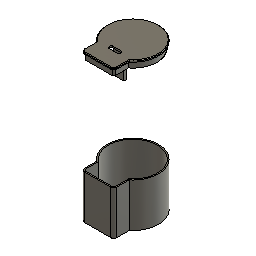
Co2SensorEnclosure (Autodesk Fusion 360 design; units mm, degrees)
Autodesk Fusion 360 part; units mm, degrees
sketch "Sketch1" plane through (0, 0, 0) normal (0, 1, 0) x (1, 0, 0)
  line L0 (0, 19) -> (0, -26.75) construction
  line L1 (0, -26.75) -> (11.5, -26.75) construction
  line L2 (10.5, -26.75) -> (-10.5, -26.75) construction
  line L3 (-11.5, -25.75) -> (-11.5, -15.1245) construction
  line L4 (11.5, -25.75) -> (11.5, -15.1245) construction
  arc A0 (-11.5, -25.75) -> (-10.5, -26.75) centre (-10.5, -25.75) ccw construction
  arc A1 (10.5, -26.75) -> (11.5, -25.75) centre (10.5, -25.75) ccw construction
  arc A2 (11.5, -15.1245) -> (-11.5, -15.1245) centre (0, 0) ccw construction
  line L5 (0, -26.75) -> (0, -20.775) construction
  line L6 (-11.5, -20.775) -> (-9.525, -20.775) construction
  circle A3 centre (-9.525, -20.775) radius 0.975
  circle A4 centre (9.525, -20.775) radius 0.975
  circle A5 centre (0, 0) radius 17.85 construction
  line L7 (10.5, -27.25) -> (-10.5, -27.25)
  arc A6 (-12, -25.75) -> (-10.5, -27.25) centre (-10.5, -25.75) ccw
  line L8 (-12, -25.75) -> (-12, -15.3704)
  arc A7 (12, -15.3704) -> (-12, -15.3704) centre (0, 0) ccw
  line L9 (12, -25.75) -> (12, -15.3704)
  arc A8 (10.5, -27.25) -> (12, -25.75) centre (10.5, -25.75) ccw
  arc A9 (10.5, -28.25) -> (13, -25.75) centre (10.5, -25.75) ccw
  line L10 (13, -25.75) -> (13, -15.8509)
  arc A10 (13, -15.8509) -> (-13, -15.8509) centre (0, 0) ccw
  line L11 (-13, -25.75) -> (-13, -15.8509)
  arc A11 (-13, -25.75) -> (-10.5, -28.25) centre (-10.5, -25.75) ccw
  line L12 (10.5, -28.25) -> (-10.5, -28.25)
  circle A12 centre (-9.525, -20.775) radius 2
  circle A13 centre (9.525, -20.775) radius 2
  circle A14 centre (0, 0) radius 17
  circle A15 centre (9.525, -20.775) radius 0.5
  circle A16 centre (-9.525, -20.775) radius 0.5
  point P0 (-11.5, -26.75)
  dimension "d1" = 38
  dimension "d2" = 45.75
  dimension "d3" = 11.5
  dimension "d4" = 23
  dimension "d5" = 26.75
  dimension "d6" = 1
  dimension "d7" = 1
  dimension "d8" = 5.975
  dimension "d10" = 9.525
  dimension "d11" = 1.95
  dimension "d12" = 1.95
  dimension "d13" = 9.525
  dimension "d16" = 5.975
  dimension "d17" = 5.975
  dimension "d18" = 1.975
  dimension "d19" = 1.975
  dimension "d20" = 35.7
  dimension "d21" = 0.5
  dimension "d22" = -1
  dimension "d25" = 4
  dimension "d26" = 4
  dimension "d29" = 34
  dimension "d36" = 1
  dimension "d37" = 1
  constraint coincident A2.centre A5.centre
  constraint coincident L0.start A2
  constraint vertical L0
  constraint perpendicular L0 L1
  constraint parallel L1 L2
  constraint perpendicular L2 L3
  constraint perpendicular L1 L4
  constraint coincident P0 L2
  constraint coincident P0 L3
  constraint tangent L2 A0
  constraint tangent L3 A0
  constraint coincident L1.end L4
  constraint coincident L1.end L2
  constraint tangent L4 A1
  constraint tangent L2 A1
  constraint perpendicular L2 L5
  constraint coincident L3 L6.start
  constraint perpendicular L3 L6
  constraint coincident L6.end A3.centre
  constraint concentric A3 A12
  constraint concentric A4 A13
  constraint concentric A2 A14
  constraint concentric A13 A15
  constraint concentric A3 A16
  measures "d1" diameter of A2
  measures "d2" distance of L0.start L0.end
  measures "d3" distance of L0.end L1.end
  measures "d4" distance of L1.end P0
  measures "d5" distance of A2.centre L1
  measures "d6" radius of A0
  measures "d7" radius of A1
  measures "d8" distance of L0.end L5.end
  measures "d10" horizontal distance of A2.centre L6.end
  measures "d11" diameter of A3
  measures "d12" diameter of A4
  measures "d13" horizontal distance of A2.centre A4.centre
  measures "d16" distance of L2 L6.end
  measures "d17" distance of L1 A4.centre
  measures "d18" distance of L3 L6.end
  measures "d19" distance of L4 A4.centre
  measures "d20" diameter of A5
  measures "d25" diameter of A12
  measures "d26" diameter of A13
  measures "d29" diameter of A14
  measures "d36" diameter of A15
  measures "d37" diameter of A16
extrude "Extrude1" add sketch "Sketch1" against normal blind 1 contours A3 | A4 | L7 A6 L8 A7 L9 A8 | A9 L10 A10 L11 A11 L12 | A12 | A13 | A14 | A15 | A16 makes body 1
extrude "Extrude4" add sketch "Sketch1" along normal blind 2 contours A3 | A4 | A12 | A13 bodies 1
extrude "Extrude3" cut sketch "Sketch1" against normal up to surface (1 mm away) contours A14 bodies 1
chamfer "Chamfer1" distance 2 distance2 0.76 1 edges at (-15.8496, -1, 6.1475) measured on face at (-0.4235, -1, 24.4842) on bodies 1
fillet "Fillet1" radius 2 1 faces at (0.4733, -1, 25.149) on bodies 1
extrude "Extrude5" add sketch "Sketch1" along normal blind 35 contours A9 L10 A10 L11 A11 L12 bodies 1
copy_body "Body->Comp1" bodies 1 removing the originals makes body 2 in component "Component"
extrude "Extrude1'" add sketch "Sketch1" along normal blind 1.3 separate body contours A3 | A4 | L7 A6 L8 A7 L9 A8 | A9 L10 A10 L11 A11 L12 | A12 | A13 | A14 | A15 | A16 makes body 3 in component "Cover"
sketch "Sketch1 (2)" plane through (0, 1.3, 0) normal (0, 1, 0) x (-1, 0, 0) in component "Cover"
  line L0 (-13, 25.75) -> (-13, 15.8509)
  arc A0 (-13, 15.8509) -> (13, 15.8509) centre (0, 0) ccw
  line L1 (13, 15.8509) -> (13, 25.75)
  arc A1 (13, 25.75) -> (10.5, 28.25) centre (10.5, 25.75) ccw
  line L2 (10.5, 28.25) -> (-10.5, 28.25)
  arc A2 (-10.5, 28.25) -> (-13, 25.75) centre (-10.5, 25.75) ccw
  line L3 (13, 15.8509) -> (-13, 15.8509) construction
  line L4 (0, 15.8509) -> (0, 12.6509) construction
  line L5 (0, 12.6509) -> (4.5, 12.6509) construction
  line L6 (3.3, 12.6509) -> (-3.3, 12.6509)
  line L7 (-4.5, 13.8509) -> (-4.5, 14.6509)
  line L8 (-3.3, 15.8509) -> (3.3, 15.8509)
  line L9 (4.5, 14.6509) -> (4.5, 13.8509)
  arc A3 (-4.5, 13.8509) -> (-3.3, 12.6509) centre (-3.3, 13.8509) ccw
  arc A4 (3.3, 12.6509) -> (4.5, 13.8509) centre (3.3, 13.8509) ccw
  arc A5 (4.5, 14.6509) -> (3.3, 15.8509) centre (3.3, 14.6509) ccw
  arc A6 (-3.3, 15.8509) -> (-4.5, 14.6509) centre (-3.3, 14.6509) ccw
  line L10 (0, 12.6509) -> (0, 11.1509) construction
  line L11 (0, 11.1509) -> (4, 11.1509) construction
  line L12 (4, 11.1509) -> (-4, 11.1509)
  line L13 (-4, 11.1509) -> (-4, 9.1509)
  line L14 (-4, 9.1509) -> (4, 9.1509)
  line L15 (4, 9.1509) -> (4, 11.1509)
  arc A7 (11.9, 25.75) -> (10.5, 27.15) centre (10.5, 25.75) ccw
  line L16 (10.5, 27.15) -> (-10.5, 27.15)
  arc A8 (-10.5, 27.15) -> (-11.9, 25.75) centre (-10.5, 25.75) ccw
  line L17 (-11.9, 25.75) -> (-11.9, 15.3216)
  arc A9 (-11.9, 15.3216) -> (11.9, 15.3216) centre (0, 0) ccw
  line L18 (11.9, 15.3216) -> (11.9, 25.75)
  arc A10 (10.9, 25.75) -> (10.5, 26.15) centre (10.5, 25.75) ccw
  line L19 (10.5, 26.15) -> (-10.5, 26.15)
  arc A11 (-10.5, 26.15) -> (-10.9, 25.75) centre (-10.5, 25.75) ccw
  line L20 (-10.9, 25.75) -> (-10.9, 14.824)
  arc A12 (-10.9, 14.824) -> (10.9, 14.824) centre (0, 0) ccw
  line L21 (10.9, 14.824) -> (10.9, 25.75)
  point P0 (-4.5, 12.6509)
  point P1 (4.5, 15.8509)
  dimension "d44" = 3.2
  dimension "d45" = 4.5
  dimension "d46" = 9
  dimension "d47" = 3.2
  dimension "d48" = 1.2
  dimension "d49" = 1.2
  dimension "d50" = 1.2
  dimension "d51" = 1.2
  dimension "d52" = 1.5
  dimension "d53" = 4
  dimension "d54" = 8
  dimension "d55" = 2
  dimension "d62" = -1.1
  dimension "d63" = -2.1
  constraint coincident A0.end L1.start
  constraint coincident L0.end A0.start
  constraint midpoint L3 L4.start
  constraint perpendicular L3 L4
  constraint perpendicular L4 L5
  constraint horizontal L6
  constraint vertical L7
  constraint horizontal L8
  constraint vertical L9
  constraint coincident P0 L7
  constraint coincident P0 L6
  constraint tangent L7 A3
  constraint tangent L6 A3
  constraint coincident L5.end L9
  constraint coincident L5.end L6
  constraint tangent L9 A4
  constraint tangent L6 A4
  constraint coincident P1 L8
  constraint coincident P1 L9
  constraint tangent L8 A5
  constraint tangent L9 A5
  constraint tangent L7 A6
  constraint tangent L8 A6
  constraint perpendicular L6 L10
  constraint perpendicular L10 L11
  constraint horizontal L12
  constraint vertical L13
  constraint horizontal L14
  constraint vertical L15
  measures "d44" distance of L4.start L4.end
  measures "d45" distance of L4.end L5.end
  measures "d46" distance of L5.end P0
  measures "d47" distance of L5.end P1
  measures "d48" radius of A3
  measures "d49" radius of A4
  measures "d50" radius of A5
  measures "d51" radius of A6
  measures "d52" distance of L4.end L10.end
  measures "d53" distance of L10.end L11.end
  measures "d54" distance of L11.end L12.end
  measures "d55" distance of L11.end L14.end
extrude "Extrude2" cut sketch "Sketch1 (2)" against normal up to surface (1.3 mm away) contours L6 L7 L8 L9 A3 A4 A5 A6 bodies 3 in component "Cover"
extrude "Extrude3'" add sketch "Sketch1 (2)" along normal blind 20 contours L12 L13 L14 L15 bodies 3 in component "Cover"
fillet "Fillet1'" radius 5 1 edges at (0, 1.3, 9.1509) on bodies 3 in component "Cover"
extrude "Extrude4'" add sketch "Sketch1 (2)" along normal blind 5 contours A7 L16 A8 L17 A9 L18 bodies 3 in component "Cover"
chamfer "Chamfer1'" distance 0.5 distance2 0.1 1 faces at (-3.5, 6.3, 26.4833) on bodies 3 in component "Cover"
fillet "Fillet2" radius 0.5 6 edges at (0, 0, -20.5) (13, 0, 20.8004) (12.2678, 0, 27.5178) (0, 0, 28.25) (-12.2678, 0, 27.5178) (-13, 0, 20.8004) on bodies 3 in component "Cover"
move_body "Move1" bodies 3 to x (1, 0, 0) y (0, 1, 0) z (0, 0, 1) at (0, 47, 0) in component "Cover"
move_body "Move2" bodies 3 to x (-1, 0, 0) y (0, -1, 0) z (0, 0, 1) at (0, 0, 0) in component "Cover"
move_body "Move3" bodies 3 to x (1, 0, 0) y (0, 1, 0) z (0, 0, 1) at (0, 99, 0) in component "Cover"
move_body "Move4" bodies 3 to x (1, 0, 0) y (0, 1, 0) z (0, 0, 1) at (0, 66, 0) in component "Cover"
component "Component" placed x (1, 0, 0) y (0, 1, 0) z (0, 0, 1) at (0, 0, 0)
component "Cover" placed x (1, 0, 0) y (0, 1, 0) z (0, 0, 1) at (0, 0, 0) in component "Component"
equation "d3 = ( 23 / 2 ) * 1 mm"
equation "d8 = 5 mm + ( 1.95 / 2 ) * 1 mm"
equation "d16 = 5.00 mm + ( 1.95 / 2 ) * 1 mm"
equation "d17 = 5.00 mm + ( 1.95 / 2 ) * 1 mm"
equation "d18 = 1 mm + ( 1.95 / 2 ) * 1 mm"
equation "d33 = 1 mm - 0.24 mm"
named bodies: "Cover"
